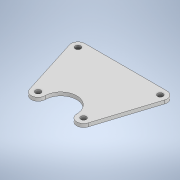
# Autodesk Inventor part: front mount base
Saved by Autodesk Inventor 2020 (Build 240168000, 168)
## iProperties
Created: 2021-05-10
Part Number: front mount base
Material: Generic
Document SubType Name: Modeling
Designer: Steven
Density: 1 g/cm^3
Appearance: Default
Author: Steven
Autodesk Inventor part; units mm, degrees
ref_plane "YZ Plane" through (0, 0, 0) normal (1, 0, 0) x (0, 1, 0)
ref_plane "XZ Plane" through (0, 0, 0) normal (0, 1, 0) x (-1, 0, 0)
ref_plane "XY Plane" through (0, 0, 0) normal (0, 0, 1) x (1, 0, 0)
sketch "Sketch1" plane through (0, 0, 0) normal (0, 1, 0) x (-1, 0, 0)
  line L0 (0, 0) -> (-48, 0) construction
  line L1 (-24, 0) -> (-24, 34) construction
  line L2 (-24, 34) -> (-37.25, 34) construction
  line L3 (-24, 34) -> (-10.75, 34) construction
  circle A0 centre (-48, 0) radius 1.6
  circle A1 centre (-37.25, 34) radius 1.6
  circle A2 centre (0, 0) radius 1.6
  circle A3 centre (-10.75, 34) radius 1.6
  arc A4 (-51.8139, 1.2059) -> (-48, -4) centre (-48, 0) ccw
  arc A5 (-33.25, 34) -> (-41.0639, 35.2059) centre (-37.25, 34) ccw
  arc A6 (0, -4) -> (3.8139, 1.2059) centre (0, 0) ccw
  arc A7 (-6.9361, 35.2059) -> (-14.75, 34) centre (-10.75, 34) ccw
  arc A8 (-33.25, 34) -> (-14.75, 34) centre (-24, 34) ccw
  line L4 (0, -4) -> (-48, -4)
  line L5 (-51.8139, 1.2059) -> (-41.0639, 35.2059)
  line L6 (3.8139, 1.2059) -> (-6.9361, 35.2059)
  dimension "d0" = 48
  dimension "d1" = 34
  dimension "d2" = 13.25
  dimension "d3" = 3.2
  dimension "d4" = 3.2
  dimension "d5" = 8
  dimension "d6" = 8
  constraints: 14 end point, 10 point on circle, 9 centre point, 6 tangent, 5 coincident, 5 symmetric about line, 1 horizontal, 1 midpoint, 1 perpendicular, 1 vertical, 4 other
  measures "d0" distance of L0.start L0.end
  measures "d1" distance of L1.start L1.end
  measures "d2" distance of L1.end L2.end
  measures "d3" diameter of A0
  measures "d4" diameter of A1
  measures "d5" diameter of A4
  measures "d6" diameter of A5
extrude "Extrusion1" add sketch "Sketch1" along normal blind 2
body "Solid1"
